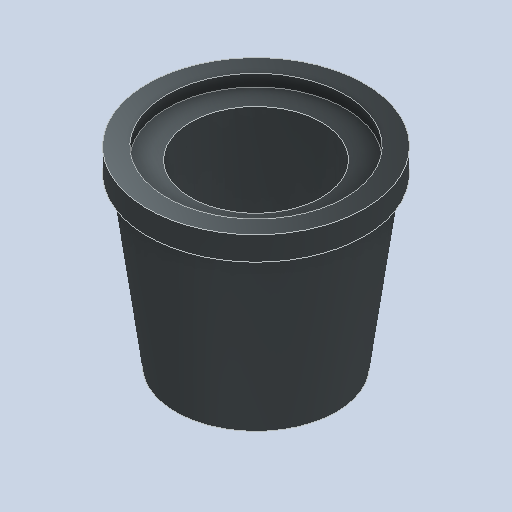
# Autodesk Inventor part: 002
Saved by Autodesk Inventor 2023 (Build 270158000, 158)
## iProperties
Created: 2022-01-03
Part Number: 002
Material: Iron, Cast
Document SubType Name: Modeling
Designer: vinicius.miguel
Density: 7.15 g/cm^3
Appearance: Iron Gray
Author: vinicius.miguel
Autodesk Inventor part; units mm, degrees
ref_plane "YZ Plane" through (0, 0, 0) normal (1, 0, 0) x (0, 1, 0)
ref_plane "XZ Plane" through (0, 0, 0) normal (0, 1, 0) x (-1, 0, 0)
ref_plane "XY Plane" through (0, 0, 0) normal (0, 0, 1) x (1, 0, 0)
sketch "Sketch1" plane through (0, 0, 0) normal (0, 0, 1) x (1, 0, 0)
  line L0 (0, 0) -> (0, -43.1) construction
  line L1 (11, 0) -> (11, -30)
  line L2 (11, -30) -> (13.5, -30)
  line L3 (13.5, -30) -> (17.25, -2)
  line L4 (18.25, 2) -> (15, 2)
  line L5 (15, 2) -> (15, 0)
  line L6 (15, 0) -> (11, 0)
  line L7 (17.25, -2) -> (18.25, -2)
  line L8 (18.25, -2) -> (18.25, 2)
  dimension "d1" = 36.5
  dimension "d2" = 22
  dimension "d3" = 30
  dimension "d4" = 2
  dimension "d5" = 1
  dimension "d6" = 30
  dimension "d7" = 27
  dimension "d8" = 2
  constraints: 18 end point, 4 perpendicular, 2 vertical, 1 horizontal, 1 horizontal alignment
  measures "d1" diameter of L8 L0
  measures "d2" diameter of L1 L0
  measures "d3" diameter of L5 L0
  measures "d4" distance of L4.end L5.end
  measures "d5" distance of L3.end L7.end
  measures "d6" distance of L1.start L1.end
  measures "d7" diameter of L2.end L0
  measures "d8" distance between parallel lines of L6 L7
revolve "Revolution1" add sketch "Sketch1" angle 360 about axis through (0, 0, 0) along (0, -1, 0)
body "Solid1"
